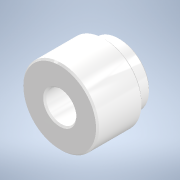
# Autodesk Inventor part: uchwyt1
Saved by Autodesk Inventor 2021 (Build 250183000, 183)
## iProperties
Created: 2021-05-20
Part Number: uchwyt1
Material: Rury z PCW
Document SubType Name: Modeling
Designer: Wojciech Wołczek
Density: 1.4 g/cm^3
Appearance: Gładki — biały
Author: Wojciech Wołczek
Autodesk Inventor part; units mm, degrees
ref_plane "YZ Plane" through (0, 0, 0) normal (1, 0, 0) x (0, 1, 0)
ref_plane "XZ Plane" through (0, 0, 0) normal (0, 1, 0) x (-1, 0, 0)
ref_plane "XY Plane" through (0, 0, 0) normal (0, 0, 1) x (1, 0, 0)
sketch "Szkic1" plane through (0, 0, 0) normal (0, 0, 1) x (1, 0, 0)
  circle A0 centre (0, 0) radius 20 projected
  circle A1 centre (0, 0) radius 20
  circle A2 centre (0, 0) radius 10
  point P0 (0, 0)
  dimension "d0" = 20
  constraints: 2 centre point, 2 coincident, 1 concentric
  measures "d0" diameter of A2
extrude "Wyciągnięcie proste1" add sketch "Szkic1" against normal blind 10
sketch "Szkic2" plane through (0, 0, 0) normal (0, 0, 1) x (1, 0, 0)
  circle A0 centre (0, 0) radius 20 projected
  circle A1 centre (0, 0) radius 10
  circle A2 centre (0, 0) radius 25
  point P0 (0, 0)
  dimension "d3" = 50
  constraints: 2 centre point, 2 coincident
  measures "d3" diameter of A2
extrude "Wyciągnięcie proste2" add sketch "Szkic2" along normal blind 30 contours A0 | A2
chamfer "Faza1" distance 1 angle 45 5 edges at (-25, 0, 0) (-20, 0, -10) (-10, 0, -10) (-25, 0, 30) (-10, 0, 30)
